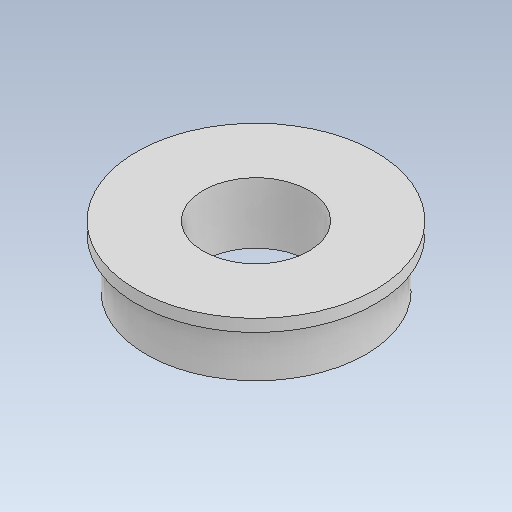
# Autodesk Inventor part: Bearing for THUNDER
Saved by Autodesk Inventor 2020 (Build 240168000, 168)
## iProperties
Created: 2020-01-15
Part Number: Bearing for THUNDER
Material: Generic
Document SubType Name: Modeling
Designer: aidan
Density: 1 g/cm^3
Appearance: Default
Author: aidan
Autodesk Inventor part; units mm, degrees
ref_plane "YZ Plane" through (0, 0, 0) normal (1, 0, 0) x (0, 1, 0)
ref_plane "XZ Plane" through (0, 0, 0) normal (0, 1, 0) x (-1, 0, 0)
ref_plane "XY Plane" through (0, 0, 0) normal (0, 0, 1) x (1, 0, 0)
sketch "Sketch2" plane through (0, 0, 0) normal (0, 0, 1) x (1, 0, 0)
  line L0 (9.9124, -0.5691) -> (9.9124, -2.1693)
  line L1 (-21.2026, -2.1693) -> (-21.2026, -0.5691)
  line L2 (8.6424, -2.1693) -> (8.6424, -8.5193)
  line L3 (-19.9326, -8.5193) -> (-19.9326, -2.1693)
  line L4 (-5.6451, 16.1255) -> (-5.6451, -16.7014) construction
  line L5 (1.2256, -0.5691) -> (1.2256, -8.5193)
  line L6 (-12.5158, -8.5193) -> (-12.5158, -0.5691)
  line L7 (9.9124, -2.1693) -> (8.6424, -2.1693)
  line L8 (-19.9326, -2.1693) -> (-21.2026, -2.1693)
  line L9 (-21.2026, -0.5691) -> (-12.5158, -0.5691)
  line L10 (1.2256, -0.5691) -> (9.9124, -0.5691)
  line L11 (8.6424, -8.5193) -> (1.2256, -8.5193)
  line L12 (-12.5158, -8.5193) -> (-19.9326, -8.5193)
  point P0 (0, 0)
  dimension "d0" = 28.575
  dimension "d1" = 31.115
  dimension "d5" = 13.7414
  constraints: 26 end point, 7 parallel, 2 horizontal, 2 perpendicular, 1 vertical, 3 other
  measures "d0" distance of L2.end L3.start
  measures "d1" distance between parallel lines of L0 L1
  measures "d5" distance between parallel lines of L5 L6
revolve "Revolution1" add sketch "Sketch2" angle 180 about axis through (-5.6451, 16.1255, 0) along (0, 1, 0)
body "Solid1"
